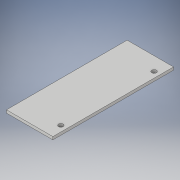
# Autodesk Inventor part: LoadCellPlate
Saved by Autodesk Inventor 2019.3 (Build 233278000, 278)
## iProperties
Created: 2019-01-26
Part Number: LoadCellPlate
Material: Generic
Document SubType Name: Modeling
Designer: mark
Density: 1 g/cm^3
Appearance: Default
Author: mark
Autodesk Inventor part; units mm, degrees
ref_plane "YZ Plane" through (0, 0, 0) normal (1, 0, 0) x (0, 1, 0)
ref_plane "XZ Plane" through (0, 0, 0) normal (0, 1, 0) x (-1, 0, 0)
ref_plane "XY Plane" through (0, 0, 0) normal (0, 0, 1) x (1, 0, 0)
sketch "Sketch1" plane through (0, 0, 0) normal (0, 1, 0) x (-1, 0, 0)
  line L0 (0, 0) -> (50.75, 0)
  line L1 (50.75, 0) -> (50.75, -132)
  line L2 (50.75, -132) -> (0, -132)
  line L3 (0, -132) -> (0, 0)
  circle A0 centre (6.275, -15) radius 2.5
  circle A1 centre (6.275, -117) radius 2.5
  dimension "d0" = 50.75
  dimension "d1" = 132
  dimension "d4" = 5
  dimension "d5" = 5
  dimension "d6" = 6.275
  dimension "d7" = 6.275
  dimension "d8" = 15
  dimension "d9" = 15
  constraints: 8 end point, 2 centre point, 2 perpendicular, 1 vertical
  measures "d0" distance of L1.end L2.end
  measures "d1" distance between parallel lines of L0 L2
  measures "d4" diameter of A0
  measures "d5" diameter of A1
  measures "d6" distance from line of L3 A0.centre
  measures "d7" distance from line of L3 A1.centre
  measures "d8" distance from line of L0 A0.centre
  measures "d9" distance from line of L2 A1.centre
extrude "Extrusion1" add sketch "Sketch1" along normal blind 3.1
body "Solid1"
